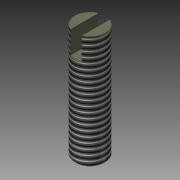
# Autodesk Inventor part: 砂轮电机皮带轮固定螺丝
Saved by Autodesk Inventor 2015 (Build 190159000, 159)
## iProperties
Created: 2017-05-24
Part Number: 砂轮电机皮带轮固定螺丝
Material: 常规
Document SubType Name: Modeling
Designer: Administrator
Density: 1 g/cm^3
Appearance: 预制平滑
Author: Administrator
Autodesk Inventor part; units mm, degrees
ref_plane "YZ Plane" through (0, 0, 0) normal (1, 0, 0) x (0, 1, 0)
ref_plane "XZ Plane" through (0, 0, 0) normal (0, 1, 0) x (-1, 0, 0)
ref_plane "XY Plane" through (0, 0, 0) normal (0, 0, 1) x (1, 0, 0)
sketch "草图1" plane through (0, 0, 0) normal (0, 0, 1) x (1, 0, 0)
  circle A0 centre (0, 0) radius 2
  dimension "d0" = 4
  constraints: 1 centre point, 1 coincident
  measures "d0" diameter of A0
extrude "拉伸1" add sketch "草图1" along normal blind 15
sketch "草图2" plane through (0, 0, 15) normal (0, 0, 1) x (1, 0, 0)
  line L0 (-0.75, 2) -> (0.75, 2)
  line L1 (0.75, 2) -> (0.75, -2)
  line L2 (0.75, -2) -> (-0.75, -2)
  line L3 (-0.75, -2) -> (-0.75, 2)
  line L4 (0, 0) -> (0, 2)
  circle A0 centre (0, 0) radius 2 projected
  dimension "d3" = 1.5
  constraints: 10 end point, 2 parallel, 2 tangent, 1 horizontal, 1 midpoint, 1 perpendicular, 1 vertical
  measures "d3" distance of L0.start L0.end
extrude "拉伸2" cut sketch "草图2" against normal blind 3 contours L0 A0 L3 | L0 L1 A0 | A0 L1 L3 | A0 L2 L3 | L1 L2 A0
thread "螺纹1" size "M4x0.7" class "6g" standard "ANSI Metric M Profile" full length
chamfer "倒角1" distance 0.25 angle 45 1 edges at (-2, 0, 0)
